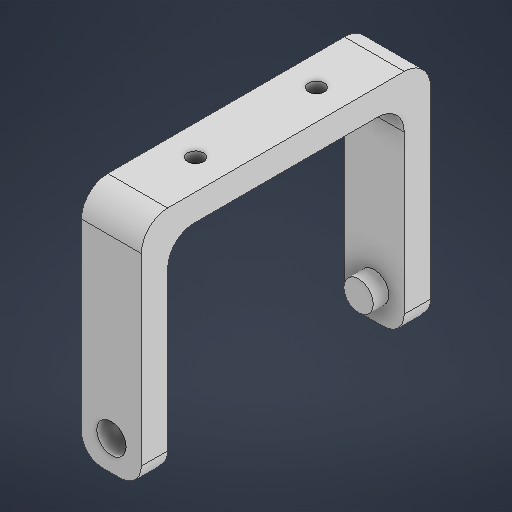
# Autodesk Inventor part: ruka_part spodni
Saved by Autodesk Inventor 2026 (Build 300175000, 175)
## iProperties
Created: 2025-04-11
Part Number: ruka_part spodni
Material: Generic
Document SubType Name: Modeling
Designer: janpa
Density: 1 g/cm^3
Appearance: Default
Author: janpa
Autodesk Inventor part; units mm, degrees
ref_plane "YZ Plane" through (0, 0, 0) normal (1, 0, 0) x (0, 1, 0)
ref_plane "XZ Plane" through (0, 0, 0) normal (0, 1, 0) x (-1, 0, 0)
ref_plane "XY Plane" through (0, 0, 0) normal (0, 0, 1) x (1, 0, 0)
sketch "Sketch2" plane through (0, 0, 0) normal (1, 0, 0) x (0, 1, 0)
  line L0 (0, 0) -> (39, 0)
  line L1 (44, -5) -> (44, -5)
  line L2 (34, -5) -> (0, -5)
  line L3 (0, -5) -> (0, 0)
  line L4 (39, -10) -> (39, -45)
  line L5 (39, -55) -> (39, -55)
  line L6 (44, -50) -> (44, -5)
  line L7 (44, -55) -> (0, -55)
  line L8 (0, -55) -> (0, -50)
  line L9 (44, -49) -> (44, -55)
  line L10 (44, -55) -> (0, -55)
  line L11 (0, -55) -> (0, -50)
  line L12 (0, -50) -> (34, -50)
  line L13 (44, -50) -> (44, -55)
  arc A0 (44, -5) -> (39, 0) centre (39, -5) ccw
  arc A1 (39, -55) -> (44, -50) centre (39, -50) ccw
  arc A2 (34, -50) -> (39, -45) centre (34, -45) ccw
  arc A3 (39, -10) -> (34, -5) centre (34, -10) ccw
  point P0 (44, 0)
  point P1 (0, -2.5)
  dimension "d12" = 44
  dimension "d13" = 50
  dimension "d14" = 5
  dimension "d16" = 5
  dimension "d17" = 5
  dimension "d18" = 39
  dimension "d19" = 5
  constraints: 28 end point, 8 point on circle, 8 tangent, 6 parallel, 4 centre point, 4 point on line, 3 equal radius, 3 horizontal, 3 perpendicular, 1 midpoint
  measures "d12" distance of L0.start point (44, 0)
  measures "d13" distance of L7.start L1.end
  measures "d14" distance of L2.end L0.start
  measures "d16" distance of L5.start L7.start
  measures "d17" distance of L8.end L10.end
  measures "d18" distance from line of point (0, -2.5) L4
  measures "d19" radius of A0
extrude "Extrusion2" add sketch "Sketch2" along normal blind 11.4 contours L0 A0 L6 A1 L7 L8 L12 A2 L4 A3 L2 L3
fillet "Fillet1" radius 4 4 edges at (11.4, 0, -2.5) (0, 0, -2.5) (11.4, 0, -52.5) (0, 0, -52.5)
sketch "Sketch3" plane through (0, 39, 0) normal (0, 0, 1) x (1, 0, 0)
  circle A0 centre (5.7, -33.3) radius 2.8
  line L0 (0, 0) -> (0, -35) projected
  line L1 (4, -39) -> (7.4, -39) projected
  point P0 (0, -39)
  point P1 (5.7, -39)
  dimension "d23" = 5.6
  dimension "d24" = 5.7
  dimension "d25" = 5.7
  constraints: 1 centre point, 1 midpoint
  measures "d23" diameter of A0
  measures "d24" distance from line of L0 A0.centre
  measures "d25" distance of point (5.7, -39) A0.centre
extrude "Extrusion3" cut sketch "Sketch3" against normal blind 11.4
sketch "Sketch4" plane through (11.4, 39, -55) normal (0, 0, -1) x (-1, 0, 0)
  circle A0 centre (5.7, -33.3) radius 2.8 projected
  circle A1 centre (5.7, -33.3) radius 2.8
  point P0 (11.4, -39)
  constraints: 1 centre point, 1 coincident
extrude "Extrusion4" add sketch "Sketch4" against normal blind 8
sketch "Sketch7" plane through (0, 39, -45) normal (0, -1, 0) x (1, 0, 0)
  circle A0 centre (5.7, 29) radius 1.5
  circle A1 centre (5.7, 6) radius 1.5
  line L0 (0, 35) -> (0, 0) projected
  line L1 (11.4, 35) -> (11.4, 0) projected
  line L2 (0, 35) -> (11.4, 35) projected
  line L3 (0, 0) -> (11.4, 0) projected
  circle A2 centre (5.7, 29) radius 2.8
  circle A3 centre (5.7, 6) radius 2.8
  point P0 (0, 45)
  dimension "d30" = 3
  dimension "d31" = 3
  dimension "d32" = 5.7
  dimension "d33" = 5.7
  dimension "d34" = 6
  dimension "d35" = 6
  dimension "d36" = 5.6
  dimension "d37" = 5.6
  constraints: 4 centre point, 2 coincident
  measures "d30" diameter of A0
  measures "d31" diameter of A1
  measures "d32" distance from line of L0 A0.centre
  measures "d33" distance from line of L1 A1.centre
  measures "d34" distance from line of L2 A0.centre
  measures "d35" distance from line of L3 A1.centre
  measures "d36" diameter of A2
  measures "d37" diameter of A3
extrude "Extrusion5" cut sketch "Sketch7" against normal blind 8 contours A0 | A1
extrude "Extrusion6" cut sketch "Sketch7" against normal blind 2 contours A2 | A3
body "Solid2"
